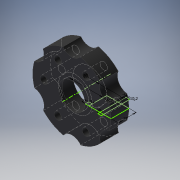
# Autodesk Inventor part: HELP_6204BEARING_CASE_A
Saved by Autodesk Inventor 2018 (Build 220112000, 112)
## iProperties
Created: 2026-07-03
Part Number: HELP_6204BEARING_CASE_A
Material: Generic
Document SubType Name: Modeling
Designer: neo
Density: 1 g/cm^3
Appearance: Default
Author: neo
Autodesk Inventor part; units mm, degrees
ref_plane "YZ Plane" through (0, 0, 0) normal (1, 0, 0) x (0, 1, 0)
ref_plane "XZ Plane" through (0, 0, 0) normal (0, 1, 0) x (-1, 0, 0)
ref_plane "XY Plane" through (0, 0, 0) normal (0, 0, 1) x (1, 0, 0)
sketch "Sketch1" plane through (0, 0, 0) normal (0, 0, 1) x (1, 0, 0)
  line L0 (-0.8746, 32.779) -> (-0.8746, -34.5944)
  line L1 (22.6254, 4.1775) -> (53.6254, 4.1775)
  line L2 (53.6254, 4.1775) -> (53.6254, -20.8225)
  line L3 (53.6254, -20.8225) -> (22.6254, -20.8225)
  line L4 (22.6254, -20.8225) -> (22.6254, 4.1775)
  line L5 (38.1254, 4.1775) -> (38.1254, -20.8225)
  line L6 (38.1254, 15.3436) -> (43.2254, 15.3436)
  line L7 (43.2254, 15.3436) -> (43.2254, -23.8453)
  line L8 (43.2254, -23.8453) -> (38.1254, -23.8453)
  line L9 (38.1254, -23.8453) -> (38.1254, 15.3436)
  line L10 (22.6254, -15.8225) -> (17.6254, -15.8225)
  line L11 (17.6254, -15.8225) -> (17.6254, -20.8225)
  line L12 (17.6254, -20.8225) -> (22.6254, -20.8225)
  line L13 (22.6254, -20.8225) -> (22.6254, -15.8225)
  point P0 (0, 0)
  dimension "d0" = 47
  dimension "d1" = 25
  dimension "d3" = 39
  dimension "d5" = 10.2
  dimension "d7" = 5
  dimension "d8" = 5
  constraints: 28 end point, 6 parallel, 3 horizontal, 3 perpendicular, 2 collinear, 2 midpoint, 1 point on line, 1 vertical
  measures "d0" diameter of L4 L0
  measures "d1" distance between parallel lines of L3 L1
  measures "d3" distance between parallel lines of L0 L5
  measures "d5" diameter of L7 L5
  measures "d7" distance of L10.start L10.end
  measures "d8" distance of L10.end L11.end
revolve "Revolution1" add sketch "Sketch1" angle 360 about axis through (-0.8746, 32.779, 0) along (0, -1, 0) contours L1 L5 L3 L4 | L1 L7 L3 L5 | L1 L2 L3 L7
revolve "Revolution2" cut sketch "Sketch1" angle 360 about axis through (38.1254, -23.8453, 0) along (0, 1, 0) contours L9 L6 L7 L1 | L1 L7 L3 L5 | L3 L7 L8 L9
revolve "Revolution3" add sketch "Sketch1" angle 360 about axis through (-0.8746, 32.779, 0) along (0, -1, 0) contours L4 L12 L11 L10
pattern_circular "Circular Pattern1" count 6 over 360 about axis through (-0.8746, -8.3225, 0) along (0, -1, 0) of "Revolution2"
sketch "Sketch2" plane through (-0.8746, -20.8225, 0) normal (0, -1, 0) x (1, 0, 0)
  circle A0 centre (-0.347, 62) radius 15
  circle A1 centre (19.5, -33.775) radius 5.1 projected
  circle A2 centre (-19.5, -33.775) radius 5.1 projected
  circle A3 centre (-39, 0) radius 5.1 projected
  circle A4 centre (-19.5, 33.775) radius 5.1 projected
  circle A5 centre (19.5, 33.775) radius 5.1 projected
  circle A6 centre (0, 0) radius 18.5 projected
  circle A7 centre (39, 0) radius 5.1 projected
  circle A8 centre (0, 0) radius 54.5 projected
  point P0 (0.8746, 0)
  dimension "d13" = 62
  dimension "d14" = 30
  constraints: 1 centre point
  measures "d13" vertical distance of A6.centre A0.centre
  measures "d14" diameter of A0
extrude "Extrusion1" cut sketch "Sketch2" against normal through all contours A0 A8 | A8 A0 picked at (-0.731, 61.8812) picked at (-0.2905, 51.8983)
pattern_circular "Circular Pattern2" count 6 over 360 about axis through (-0.8746, -8.3225, 0) along (0, -1, 0) of "Extrusion1"
body "Solid1"
